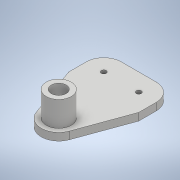
# Autodesk Inventor part: переходник2
Saved by Autodesk Inventor 2020 (Build 240168000, 168)
## iProperties
Created: 2020-01-23
Part Number: переходник2
Material: Типовые
Document SubType Name: Modeling
Designer: Css38
Density: 1 g/cm^3
Appearance: По умолчанию
Author: Css38
Autodesk Inventor part; units mm, degrees
ref_plane "YZ Plane" through (0, 0, 0) normal (1, 0, 0) x (0, 1, 0)
ref_plane "XZ Plane" through (0, 0, 0) normal (0, 1, 0) x (-1, 0, 0)
ref_plane "XY Plane" through (0, 0, 0) normal (0, 0, 1) x (1, 0, 0)
sketch "Эскиз1" plane through (0, 0, 0) normal (0, 0, 1) x (1, 0, 0)
  line L0 (-7, -3.5) -> (7, -3.5) construction
  line L1 (7, -3.5) -> (7, 3.5)
  line L2 (7, 3.5) -> (-7, 3.5)
  line L3 (-7, 3.5) -> (-7, -3.5)
  line L4 (-7, -3.5) -> (7, 3.5) construction
  line L5 (7, -3.5) -> (-7, 3.5) construction
  line L6 (0, -3.5) -> (0, -12.5) construction
  line L7 (-7, -3.5) -> (-3.289, -13.697)
  line L8 (7, -3.5) -> (3.289, -13.697)
  arc A0 (-3.289, -13.697) -> (3.289, -13.697) centre (0, -12.5) ccw
  point P0 (0, 0)
  point P1 (0, 0)
  point P2 (0, 0)
  point P3 (0, 0)
  dimension "d0" = 14
  dimension "d1" = 7
  dimension "d4" = 9
  dimension "d5" = 3.5
  constraints: 18 end point, 3 coincident, 3 midpoint, 2 parallel, 2 point on circle, 1 centre point, 1 equal length, 1 horizontal, 1 perpendicular, 1 tangent, 1 vertical
  measures "d0" distance of L2.end L1.end
  measures "d1" distance of L0.end L1.end
  measures "d4" distance of L6.start L6.end
  measures "d5" radius of A0
extrude "Выдавливание1" add sketch "Эскиз1" along normal blind 1.5
sketch "Эскиз2" plane through (0, 0, 1.5) normal (0, 0, 1) x (1, 0, 0)
  arc A0 (-3.289, -13.697) -> (3.289, -13.697) centre (0, -12.5) ccw construction
  circle A1 centre (0, -12.5) radius 2.5
  circle A2 centre (0, -12.5) radius 1.5
  point P0 (0, 0)
  dimension "d8" = 5
  dimension "d39" = 1
  constraints: 2 centre point, 1 coincident
  measures "d8" diameter of A1
  measures "d39" radial gap between concentric circles of A1 A2
extrude "Выдавливание11" add sketch "Эскиз2" along normal blind 5
fillet "Сопряжение1" radius 3.5 2 edges at (7, 3.5, 0.75) (-7, 3.5, 0.75)
sketch "Эскиз5" plane through (0, 0, 0) normal (0, 0, 1) x (1, 0, 0)
  circle A0 centre (0, -12.5) radius 1.25 construction
  line L0 (0, -3.5) -> (0, 3.5) construction
  circle A1 centre (3.5, 0) radius 0.5
  line L1 (3.5, 0) -> (3.5, 3.5) construction
  line L2 (3.5, 0) -> (0, 0) construction
  line L3 (3.5, 3.5) -> (-3.5, 3.5) construction
  circle A2 centre (-3.5, 0) radius 0.5
  point P0 (-7, 3.5)
  point P1 (7, -3.5)
  point P2 (7, 3.5)
  dimension "d34" = 1
  dimension "d35" = 3.5
  constraints: 7 end point, 2 centre point, 2 midpoint, 2 perpendicular, 2 vertical, 1 horizontal alignment, 1 symmetric about line, 1 other
  measures "d34" diameter of A1
  measures "d35" distance of L1.start L1.end
hole "Отверстие1" at (-3.5, 0, 0) at (3.5, 0, 0) direction (0, 0, 1) diameter 1 end through all countersink diameter 1.5 countersink angle 90
